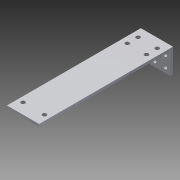
# Autodesk Inventor part: Flange for 3-4 in Piston
Saved by Autodesk Inventor 2014 (Build 180170000, 170)
## iProperties
Created: 2014-01-05
Part Number: Flange for 3-4 in Piston
Material: Aluminum
Document SubType Name: Sheet Metal
Designer: Michael
Density: 2.71 g/cm^3
Sheet Metal Rule: Default
Appearance: Satin
Author: Michael
Autodesk Inventor part; units mm, degrees
ref_plane "YZ Plane" through (0, 0, 0) normal (1, 0, 0) x (0, 1, 0)
ref_plane "XZ Plane" through (0, 0, 0) normal (0, 1, 0) x (-1, 0, 0)
ref_plane "XY Plane" through (0, 0, 0) normal (0, 0, 1) x (1, 0, 0)
sketch "Sketch1" plane through (0, 0, 0) normal (0, 0, 1) x (1, 0, 0)
  line L0 (0, 0) -> (38.1, 0)
  line L1 (38.1, 0) -> (38.1, 25.4)
  line L2 (38.1, 25.4) -> (0, 25.4)
  line L3 (0, 25.4) -> (0, 0)
  circle A0 centre (6.35, 6.35) radius 2.4892
  circle A1 centre (6.35, 19.05) radius 2.4892
  circle A2 centre (19.05, 6.35) radius 2.4892
  circle A3 centre (19.05, 19.05) radius 2.4892
  circle A4 centre (31.75, 6.35) radius 2.4892
  circle A5 centre (31.75, 19.05) radius 2.4892
  dimension "d0" = 38.1
  dimension "d1" = 25.4
  dimension "d2" = 4.9784
  dimension "d3" = 6.35
  dimension "d4" = 6.35
  dimension "d7" = 12.7
  dimension "d10" = 12.7
  measures "d0" distance of L2.end L1.end
  measures "d1" distance of L1.end L0.end
  measures "d2" diameter of A0
  measures "d3" distance from line of L0 A0.centre
  measures "d4" distance from line of L3 A0.centre
  measures "d7" distance of A0.centre A1.centre
  measures "d10" distance of A0.centre A2.centre
extrude "Plate1" add sketch "Sketch1" along normal blind 3.175
sketch "Sketch2" plane through (0, 25.4, 0) normal (0, 1, 0) x (1, 0, 0)
  line L0 (0, -3.175) -> (38.1, -3.175) projected
  line L1 (38.1, 0) -> (38.1, -3.175) projected
  line L2 (0, 0) -> (38.1, 0)
  line L3 (38.1, 0) -> (38.1, -158.75)
  line L4 (38.1, -158.75) -> (0, -158.75)
  line L5 (0, -158.75) -> (0, 0)
  circle A0 centre (6.35, -146.05) radius 2.4384
  line L6 (19.05, -158.75) -> (19.05, -3.175) construction
  circle A1 centre (31.75, -146.05) radius 2.4384
  circle A2 centre (7.6581, -23.6982) radius 2.4384
  circle A3 centre (7.6581, -10.9982) radius 2.4384
  circle A4 centre (30.4419, -23.6982) radius 2.4384
  circle A5 centre (30.4419, -10.9982) radius 2.4384
  line L7 (7.6581, -10.9982) -> (7.6581, -23.6982) construction
  dimension "d14" = 4.8768
  dimension "d15" = 158.75
  dimension "d16" = 12.7
  dimension "d17" = 12.7
  dimension "d21" = 12.7
  dimension "d22" = 11.3919
  dimension "d23" = 122.3518
  constraints: 12 end point, 6 centre point, 3 symmetric about line, 2 equal radius, 2 midpoint, 2 parallel, 1 collinear, 1 horizontal, 1 perpendicular, 1 vertical, 3 other
  measures "d14" diameter of A0
  measures "d15" distance of L4.end L2.start
  measures "d16" distance from line of L6 A0.centre
  measures "d17" distance from line of L4 A0.centre
  measures "d21" distance of L7.end L7.start
  measures "d22" distance from line of L6 L7.end
  measures "d23" vertical distance of L7.end A0.centre
extrude "Extrusion1" add sketch "Sketch2" along normal blind 3.175
equation "\"BendRadius\" = Thickness"
equation "\"BendReliefWidth\" = Thickness"
equation "\"BendReliefDepth\" = 0.5 * Thickness"
equation "\"CornerReliefSize\" = 4 * Thickness"
equation "\"MinimumRemnant\" = 2 * Thickness"
equation "\"TransitionRadius\" = BendRadius"
equation "\"JacobiRadiusSize\" = BendRadius"
equation "\"GapSize\" = Thickness"
equation "\"d13\" = BendRadius"
equation "\"Thickness\" = 3.175"
body "Solid1"
